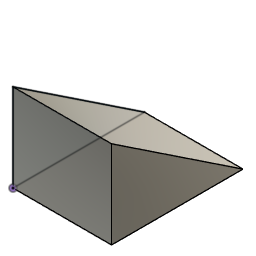
Bit (Autodesk Fusion 360 design; units mm, degrees)
Autodesk Fusion 360 part; units mm, degrees
sketch "Sketch1" plane through (0, 0, 0) normal (1, 0, 0) x (0, 1, 0)
  line L0 (0, 0) -> (0, 15.24)
  line L1 (0, 15.24) -> (22.86, 0)
  line L2 (0, 0) -> (22.86, 0)
  dimension "d3" = 15.24
  dimension "d4" = 22.86
  constraint coincident L0.start L2.start
  constraint vertical L0
  constraint perpendicular L0 L2
  measures "d3" distance of L0.start L0.end
  measures "d4" distance of L0.start L1.end
extrude "Extrude1" add sketch "Sketch1" along normal blind 17.145
equation "heightToPush = 0.6 in"
equation "width = 0.9 in"
equation "d3 = heightToPush"
equation "d4 = width"
equation "thickness = ReaderThickness * 3 / 4"
equation "d6 = thickness"
equation "ReaderThickness = 0.9 in"
